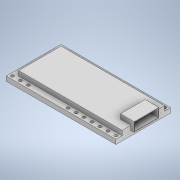
# Autodesk Inventor part: Teensy 3.2
Saved by Autodesk Inventor 2022 (Build 260153000, 153)
## iProperties
Created: 2021-10-21
Part Number: Teensy 3.2
Material: Generic
Document SubType Name: Modeling
Designer: kylem
Density: 1 g/cm^3
Appearance: Default
Author: kylem
Autodesk Inventor part; units mm, degrees
ref_plane "YZ Plane" through (0, 0, 0) normal (1, 0, 0) x (0, 1, 0)
ref_plane "XZ Plane" through (0, 0, 0) normal (0, 1, 0) x (-1, 0, 0)
ref_plane "XY Plane" through (0, 0, 0) normal (0, 0, 1) x (1, 0, 0)
sketch "Sketch1" plane through (0, 0, 0) normal (0, 1, 0) x (-1, 0, 0)
  line L0 (0, 0) -> (35.56, 0)
  line L1 (35.56, 0) -> (35.56, -17.75)
  line L2 (35.56, -17.75) -> (0, -17.75)
  line L3 (0, -17.75) -> (0, 0)
  dimension "d0" = 35.56
  dimension "d1" = 17.75
  constraints: 8 end point, 2 parallel, 1 horizontal, 1 perpendicular
  measures "d0" distance of L1.end L2.end
  measures "d1" distance of L0.end L1.end
extrude "Extrusion1" add sketch "Sketch1" along normal blind 1.5
sketch "Sketch2" plane through (0, 1.5, 0) normal (0, 1, 0) x (1, 0, 0)
  line L0 (0, 0) -> (0, 17.75) projected
  line L1 (0, 0) -> (0, 2)
  line L2 (-35.56, 17.75) -> (-35.56, 0) projected
  line L3 (-35.56, 0) -> (-33.56, 0)
  line L4 (-33.56, 0) -> (-33.56, 2)
  line L5 (-33.56, 2) -> (-35.56, 2)
  line L6 (-35.56, 2) -> (-35.56, 0)
  line L7 (0, 17.75) -> (-35.56, 17.75) projected
  line L8 (-35.56, 17.75) -> (-33.56, 17.75)
  line L9 (-33.56, 17.75) -> (-33.56, 15.75)
  line L10 (-33.56, 15.75) -> (-35.56, 15.75)
  line L11 (-35.56, 15.75) -> (-35.56, 17.75)
  line L12 (0, 17.75) -> (0, 15.75)
  line L13 (0, 15.75) -> (-33.56, 15.75)
  line L14 (-33.56, 2) -> (-33.56, 15.75)
  line L15 (-33.56, 2) -> (0, 2)
  dimension "d4" = 2
  dimension "d5" = 2
  dimension "d6" = 2
  dimension "d7" = 2
  dimension "d8" = 2
  dimension "d9" = 2
  constraints: 26 end point, 4 parallel, 2 horizontal, 2 perpendicular, 2 point on line
  measures "d4" distance of L0.start L1.end
  measures "d5" distance of L5.end L4.end
  measures "d6" distance of L4.end L3.end
  measures "d7" distance of L9.end L10.end
  measures "d8" distance of L8.end L9.end
  measures "d9" distance of L0.end L12.end
extrude "Extrusion2" add sketch "Sketch2" along normal blind 1.5 contours L15 L14 L13 L0
sketch "Sketch3" plane through (0, 0, 0) normal (1, 0, 0) x (0, 0, -1)
  line L0 (0, 0) -> (0, 1.5) projected
  line L1 (0, 1.5) -> (17.75, 1.5)
  line L2 (2, 1.5) -> (15.75, 1.5) projected
  line L3 (8.875, 1.5) -> (12.875, 1.5)
  line L4 (12.875, 1.5) -> (4.875, 1.5)
  line L5 (4.875, 1.5) -> (4.875, 4.5)
  line L6 (4.875, 4.5) -> (12.875, 4.5)
  line L7 (12.875, 4.5) -> (12.875, 1.5)
  dimension "d12" = 4
  dimension "d13" = 8
  dimension "d14" = 3
  constraints: 12 end point, 2 parallel, 1 horizontal, 1 midpoint, 1 perpendicular, 1 point on line
  measures "d12" distance of L3.start L3.end
  measures "d13" distance of L5.end L6.end
  measures "d14" distance of L4.end L5.end
extrude "Extrusion3" add sketch "Sketch3" along normal blind 1
sketch "Sketch4" plane through (0, 0, 0) normal (-1, 0, 0) x (0, 0, 1)
  line L0 (-12.875, 3) -> (-12.875, 4.5) projected
  line L1 (-4.875, 4.5) -> (-4.875, 1.5) projected
  line L2 (-12.875, 4.5) -> (-4.875, 4.5)
  line L3 (-4.875, 4.5) -> (-4.875, 3)
  line L4 (-4.875, 3) -> (-12.875, 3)
  line L5 (-12.875, 3) -> (-12.875, 4.5)
  point P0 (0, 0)
  constraints: 8 end point, 2 parallel, 1 horizontal, 1 midpoint, 1 perpendicular
extrude "Extrusion4" add sketch "Sketch4" along normal blind 3.4
sketch "Sketch5" plane through (1, 0, 0) normal (1, 0, 0) x (0, 0, -1)
  line L0 (4.875, 4.5) -> (4.875, 1.5) projected
  line L1 (4.875, 4.5) -> (5.075, 4.5)
  line L2 (5.075, 4.5) -> (5.075, 4.3)
  line L3 (5.075, 4.3) -> (4.875, 4.3)
  line L4 (4.875, 4.3) -> (4.875, 4.5)
  line L5 (12.875, 1.5) -> (12.875, 4.5) projected
  line L6 (12.875, 1.5) -> (12.675, 1.5)
  line L7 (12.675, 1.5) -> (12.675, 1.7)
  line L8 (12.675, 1.7) -> (12.875, 1.7)
  line L9 (12.875, 1.7) -> (12.875, 1.5)
  line L10 (12.675, 1.7) -> (5.075, 1.7)
  line L11 (5.075, 1.7) -> (5.075, 4.3)
  line L12 (5.075, 4.3) -> (12.675, 4.3)
  line L13 (12.675, 4.3) -> (12.675, 1.7)
  point P0 (0, 0)
  dimension "d19" = 0.2
  dimension "d20" = 0.2
  dimension "d21" = 0.2
  dimension "d22" = 0.2
  constraints: 24 end point, 6 parallel, 3 horizontal, 3 perpendicular
  measures "d19" distance of L2.end L3.end
  measures "d20" distance of L1.end L2.end
  measures "d21" distance of L7.end L8.end
  measures "d22" distance of L6.end L7.end
extrude "Extrusion5" cut sketch "Sketch5" against normal blind 4 contours L12 L13 L10 L11
sketch "Sketch6" plane through (0, 1.5, 0) normal (0, 1, 0) x (1, 0, 0)
  line L0 (0, 0) -> (0, 17.75) projected
  line L1 (0, 0) -> (0, 1)
  line L2 (0, 1) -> (-1, 1)
  circle A0 centre (-1, 1) radius 0.5
  circle A1 centre (-3.5815, 1) radius 0.5
  circle A2 centre (-6.1631, 1) radius 0.5
  circle A3 centre (-8.7446, 1) radius 0.5
  circle A4 centre (-11.3262, 1) radius 0.5
  circle A5 centre (-13.9077, 1) radius 0.5
  circle A6 centre (-16.4892, 1) radius 0.5
  circle A7 centre (-19.0708, 1) radius 0.5
  circle A8 centre (-21.6523, 1) radius 0.5
  circle A9 centre (-24.2339, 1) radius 0.5
  circle A10 centre (-26.8154, 1) radius 0.5
  circle A11 centre (-29.3969, 1) radius 0.5
  circle A12 centre (-31.9785, 1) radius 0.5
  circle A13 centre (-34.56, 1) radius 0.5
  line L3 (-35.56, 0) -> (0, 0) projected
  line L4 (0, 17.75) -> (-35.56, 17.75) projected
  line L5 (-35.56, 0) -> (-35.56, 17.75)
  line L6 (-35.56, 17.75) -> (-35.56, 0) projected
  line L7 (-35.56, 8.875) -> (-37.649, 8.875)
  line L8 (0, 17.75) -> (0, 0)
  line L9 (0, 17.75) -> (0, 16.75)
  line L10 (0, 16.75) -> (-1, 16.75)
  circle A14 centre (-1, 16.75) radius 0.5
  circle A15 centre (-3.5815, 16.75) radius 0.5
  circle A16 centre (-6.1631, 16.75) radius 0.5
  circle A17 centre (-8.7446, 16.75) radius 0.5
  circle A18 centre (-11.3262, 16.75) radius 0.5
  circle A19 centre (-13.9077, 16.75) radius 0.5
  circle A20 centre (-16.4892, 16.75) radius 0.5
  circle A21 centre (-19.0708, 16.75) radius 0.5
  circle A22 centre (-21.6523, 16.75) radius 0.5
  circle A23 centre (-24.2339, 16.75) radius 0.5
  circle A24 centre (-26.8154, 16.75) radius 0.5
  circle A25 centre (-29.3969, 16.75) radius 0.5
  circle A26 centre (-31.9785, 16.75) radius 0.5
  circle A27 centre (-34.56, 16.75) radius 0.5
  line L11 (-35.56, 17.75) -> (0, 17.75)
  dimension "d25" = 1
  dimension "d26" = 1
  dimension "d27" = 1
  dimension "d30" = 2.5815
  constraints: 28 centre point, 18 symmetric about line, 16 end point, 2 coincident, 2 horizontal, 2 point on line, 1 midpoint, 1 perpendicular, 1 vertical, 40 other
  measures "d25" distance of L0.start L1.end
  measures "d26" distance of L1.end L2.end
  measures "d27" diameter of A0
  measures "d30" distance of A0.centre A1.centre
extrude "Extrusion6" cut sketch "Sketch6" against normal blind 4 contours A0 | A14 | A1 | A2 | A3 | A4 | A5 | A6 | A7 | A8 | A9 | A10 | A11 | A12 | A13 | A15 | A16 | A17 | A18 | A19 | A20 | A21 | A22 | A23 | A24 | A25 | A26 | A27
sketch "Sketch7" plane through (0, 1.5, 0) normal (0, 1, 0) x (1, 0, 0)
  line L0 (0, 2) -> (-33.56, 2) projected
  line L1 (-27.8322, 0.2614) -> (-18.3502, 0.2614)
  line L2 (-18.3502, 0.2614) -> (-18.3502, 2)
  line L3 (-18.3502, 2) -> (-27.8322, 2)
  line L4 (-27.8322, 2) -> (-27.8322, 0.2614)
  point P0 (0, 0)
  constraints: 8 end point, 2 parallel, 1 horizontal, 1 perpendicular, 1 point on line
extrude "Extrusion7" add sketch "Sketch7" against normal blind 1.5
body "Solid1"
